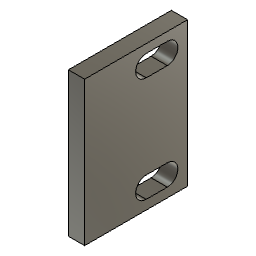
BeelinkRackmount v1 (Autodesk Fusion 360 design; units mm, degrees)
Autodesk Fusion 360 part; units mm, degrees
note: some values were not read from the file. Set by a fixed rule: which sketch regions a step uses.
sketch "Sketch1" plane through (0, 0, 0) normal (1, 0, 0) x (0, 1, 0) in component "Wing"
  line L0 (0, 0) -> (31.75, 0)
  line L1 (31.75, 0) -> (31.75, 44.45)
  line L2 (31.75, 44.45) -> (0, 44.45)
  line L3 (0, 44.45) -> (0, 0)
  dimension "d1" = 31.75
  dimension "d2" = 44.45
  constraint horizontal L0
  constraint vertical L1
  constraint horizontal L2
  constraint vertical L3
  constraint coincident L0.start L3.end
  measures "d1" distance of L0.start L0.end
  measures "d2" distance of L0.start L2.end
extrude "Extrude1" add sketch "Sketch1" against normal blind 5 makes body 1 in component "Wing"
sketch "Sketch3" plane through (-5, 0, 0) normal (-1, 0, 0) x (0, -1, 0) in component "Wing"
  line L0 (0, 0) -> (0, 44.45)
  line L1 (0, 44.45) -> (-31.75, 44.45)
  line L2 (-31.75, 44.45) -> (-31.75, 0)
  line L3 (-31.75, 0) -> (0, 0)
  line L4 (-25.497, 41.8155) -> (-18.997, 41.8155)
  line L5 (-18.997, 41.8155) -> (-18.997, 35.3155)
  line L6 (-18.997, 35.3155) -> (-25.497, 35.3155)
  line L7 (-25.497, 35.3155) -> (-25.497, 41.8155)
  circle A0 centre (-18.997, 38.5655) radius 3.25
  circle A1 centre (-25.497, 38.5655) radius 3.25
  dimension "d13" = 6.5
  dimension "d14" = 6.5
  dimension "d15" = 6.5
  dimension "d16" = 6.5
  constraint horizontal L4
  constraint vertical L5
  constraint horizontal L6
  constraint vertical L7
  constraint midpoint L5 A0.centre
  constraint midpoint L7 A1.centre
  measures "d13" distance of L4.start L4.end
  measures "d14" distance of L4.start L6.end
  measures "d15" diameter of A0
  measures "d16" diameter of A1
extrude "Extrude2" add sketch "Sketch3" against normal blind 5 separate body contours L7 A1 | L4 A0 A1 | L7 A1 | L5 A0 | L5 A0 | L6 A0 A1 makes body 2 in component "Wing"
copy_body "CopyPasteBodies1" bodies 2 makes body 3 in component "Wing"
move_body "Move1" bodies 3 to x (1, 0, 0) y (0, 1, 0) z (0, 0, 1) at (0, 0, -35.25) in component "Wing"
move_body "Move2" bodies 3 to x (1, 0, 0) y (0, 1, 0) z (0, 0, 1) at (0, 0, 2.8) in component "Wing"
combine "Combine1" operation cut target body 1 tool bodies 2 3 in component "Wing"
component "Wing" placed x (1, 0, 0) y (0, 1, 0) z (0, 0, 1) at (0, 0, 0)
